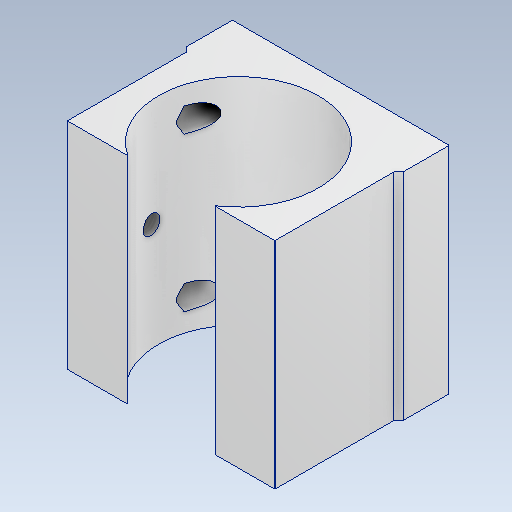
# Autodesk Inventor part: Soporte de Motor
Saved by Autodesk Inventor 2020 (Build 240168000, 168)
## iProperties
Created: 2020-06-05
Part Number: Soporte de Motor
Material: Aluminio 6061
Document SubType Name: Modeling
Designer: Pipi
Density: 2.7 g/cm^3
Appearance: Aluminio - Plano
Author: Pipi
Autodesk Inventor part; units mm, degrees
ref_plane "YZ Plane" through (0, 0, 0) normal (1, 0, 0) x (0, 1, 0)
ref_plane "XZ Plane" through (0, 0, 0) normal (0, 1, 0) x (-1, 0, 0)
ref_plane "XY Plane" through (0, 0, 0) normal (0, 0, 1) x (1, 0, 0)
sketch "Boceto1" plane through (0, 0, 0) normal (0, 1, 0) x (-1, 0, 0)
  line L0 (10.2901, 15.6998) -> (10.2901, -54.8002)
  line L1 (10.2901, -54.8002) -> (-6.2099, -54.8002)
  line L2 (-44.9099, -53.3002) -> (-44.9099, 14.1998)
  line L3 (-6.2099, 15.6998) -> (10.2901, 15.6998)
  line L4 (10.2901, 15.6998) -> (-6.2099, 15.6998)
  line L5 (-6.2099, 15.6998) -> (-6.2099, 14.1998)
  line L6 (-6.2099, 14.1998) -> (-44.9099, 14.1998)
  line L7 (10.2901, -54.8002) -> (-6.2099, -54.8002)
  line L8 (-6.2099, -54.8002) -> (-6.2099, -53.3002)
  line L9 (-6.2099, -53.3002) -> (-44.9099, -53.3002)
  circle A0 centre (-23.0099, -19.5502) radius 26
  point P0 (0, 0)
  point P1 (-44.9099, -5.5363)
  point P2 (-44.9099, -33.5641)
  dimension "d0" = 70.5
  dimension "d3" = 16.5
  dimension "d4" = 1.5
  dimension "d5" = 1.5
  dimension "d6" = 55.2
  dimension "d7" = 67.5
  dimension "d8" = 52
  dimension "d9" = 33.3
  dimension "d10" = 33.75
  constraints: 20 end point, 5 perpendicular, 2 point on line, 1 centre point, 1 vertical
  measures "d0" distance of L0.start L0.end
  measures "d3" distance of L3.start L0.start
  measures "d4" distance of L3.start L5.end
  measures "d5" distance of L1.end L8.end
  measures "d6" distance between parallel lines of L2 L0
  measures "d7" distance between parallel lines of L9 L6
  measures "d8" diameter of A0
  measures "d9" distance from line of L0 A0.centre
  measures "d10" distance from line of L9 A0.centre
extrude "Extrusión1" add sketch "Boceto1" along normal blind 70 contours L0 L1 L8 L9 L2 A0 L6 L5 L3
fillet "Empalme1" radius 0.25 2 edges at (-10.2901, 35, 15.6998) (-10.2901, 35, -54.8002)
chamfer "Chaflán1" distance 1.5 angle 45 1 edges at (6.2099, 35, 15.6998)
chamfer "Chaflán2" distance 1.5 angle 45 1 edges at (6.2099, 35, -54.8002)
sketch "Boceto2" plane through (-10.2901, 0, -54.5502) normal (-1, 0, 0) x (0, 0, 1)
  line L0 (9, 70) -> (61, 70) projected
  line L1 (35, 70) -> (35, 0)
  line L2 (0, 0) -> (70, 0) projected
  line L3 (35, 35) -> (-0.338, 35)
  line L4 (-0.338, 35) -> (70.438, 35)
  line L5 (35, 35) -> (59.975, 35)
  line L6 (35, 35) -> (10, 35)
  line L7 (10, 35) -> (10, 60)
  line L8 (10, 60) -> (60, 60)
  line L9 (60, 60) -> (60, 10)
  line L10 (60, 10) -> (10, 10)
  line L11 (10, 10) -> (10, 60)
  circle A0 centre (10, 60) radius 4
  circle A1 centre (60, 60) radius 4
  circle A2 centre (10, 10) radius 4
  circle A3 centre (60, 10) radius 4
  circle A4 centre (35, 35) radius 2
  point P0 (54.5502, 0)
  point P1 (49.0139, 70)
  point P2 (20.9861, 70)
  dimension "d23" = 25
  dimension "d24" = 50
  dimension "d25" = 50
  dimension "d26" = 8
  dimension "d27" = 8
  dimension "d28" = 8
  dimension "d29" = 8
  dimension "d30" = 4
  dimension "d73" = 25
  constraints: 20 end point, 5 centre point, 5 coincident, 3 midpoint, 3 point on line, 2 horizontal, 2 parallel, 2 perpendicular
  measures "d23" distance of L6.end L7.end
  measures "d24" distance of L9.end L10.end
  measures "d25" distance between parallel lines of L10 L8
  measures "d26" diameter of A0
  measures "d27" diameter of A1
  measures "d28" diameter of A2
  measures "d29" diameter of A3
  measures "d30" diameter of A4
  measures "d73" distance between parallel lines of L11 L1
hole "Agujero1" at (-10.2901, 60, -44.5502) at (-10.2901, 60, 5.4498) at (-10.2901, 10, -44.5502) at (-10.2901, 10, 5.4498) direction (1, 0, 0) diameter 8 depth 26 tip angle 118
thread "Rosca1" size "M8x1.25" class "6H" standard "ISO Metric profile" length 11.5
thread "Rosca2" size "M8x1.25" class "6H" standard "ISO Metric profile" length 11.5
thread "Rosca3" size "M8x1.25" class "6H" standard "ISO Metric profile" length 11.5
thread "Rosca4" size "M8x1.25" class "6H" standard "ISO Metric profile" length 11.5
hole "Agujero2" at (-10.2901, 35, -19.5502) direction (1, 0, 0) diameter 4 depth 26 tip angle 118
thread "Rosca5" size "M4x0.7" class "6H" standard "ISO Metric profile" length 11.5
chamfer "Chaflán3" distance 0.25 angle 45 5 edges at (-10.2901, 60, -48.5502) (-10.2901, 60, 1.4498) (-10.2901, 10, -48.5502) (-10.2901, 10, 1.4498) (-10.2901, 35, -21.5502)
sketch "Boceto3" plane through (44.9099, 0, 14.1998) normal (0, 0, 1) x (1, 0, 0)
  point P0 (-44.9099, 0)
sketch "Boceto4" plane through (44.9099, 0, 14.1998) normal (0, 0, 1) x (1, 0, 0)
  line L0 (-38.7, 0) -> (-38.7, 70) projected
  line L1 (-38.7, 0) -> (-38.7, 70)
  line L2 (-47.9, 70) -> (0, 70) projected
  line L3 (-38.7, 70) -> (0, 70)
  line L4 (0, 0) -> (0, 70) projected
  line L5 (0, 70) -> (0, 0)
  line L6 (0, 0) -> (-38.7, 0)
  line L7 (-47.9, 0) -> (0, 0) projected
  line L8 (-19.35, 0) -> (-19.35, 70)
  line L9 (-19.35, 35) -> (-14.4981, 35)
  line L10 (-14.4981, 35) -> (-25.37, 35)
  circle A0 centre (-19.35, 35) radius 3
  point P0 (-44.9099, 0)
  dimension "d58" = 6
  constraints: 14 end point, 2 collinear, 2 midpoint, 2 perpendicular, 2 point on line, 1 centre point, 1 coincident, 1 horizontal
  measures "d58" diameter of A0
hole "Agujero3" at (25.5599, 35, 14.1998) direction (0, 0, -1) diameter 6 depth 26 tip angle 118
thread "Rosca6" size "M6x1" class "6H" standard "ISO Metric profile" length 11.5
chamfer "Chaflán4" distance 0.25 angle 45 1 edges at (25.5599, 38, 14.1998)
fillet "Empalme2" radius 0.1 2 edges at (44.9099, 35, -5.5363) (44.9099, 35, -33.5641)
fillet "Empalme3" radius 0.2 2 edges at (44.9099, 35, -53.3002) (44.9099, 35, 14.1998)
